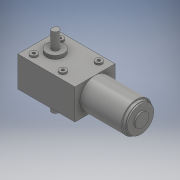
# Autodesk Inventor part: GEARBOX PURNIMA SAMARARATNE
Saved by Autodesk Inventor 2018 (Build 220112000, 112)
## iProperties
Created: 2018-06-19
Part Number: GEARBOX PURNIMA SAMARARATNE
Material: Steel
Document SubType Name: Modeling
Designer: m227958
Density: 7.85 g/cm^3
Appearance: Plate
Author: m227958
Autodesk Inventor part; units mm, degrees
ref_plane "YZ Plane" through (0, 0, 0) normal (1, 0, 0) x (0, 1, 0)
ref_plane "XZ Plane" through (0, 0, 0) normal (0, 1, 0) x (-1, 0, 0)
sketch "Sketch1" plane through (0, 0, 0) normal (1, 0, 0) x (0, 1, 0)
  line L0 (29, 22) -> (-29, 22)
  line L1 (-29, 22) -> (-29, -22)
  line L2 (-29, -22) -> (29, -22)
  line L3 (29, -22) -> (29, 22)
  dimension "d4" = 58
  dimension "d5" = 44
  constraints: 8 end point, 2 parallel, 1 horizontal, 1 perpendicular
  measures "d4" distance of L2.end L1.end
  measures "d5" distance of L1.end L0.end
extrude "Extrusion1" add sketch "Sketch1" along normal blind 82.5
sketch "Sketch2" plane through (82.5, 0, 0) normal (1, 0, 0) x (0, 0, -1)
  circle A0 centre (0, 0) radius 22
  dimension "d8" = 44
  constraints: 1 centre point, 1 coincident
  measures "d8" diameter of A0
extrude "Extrusion2" add sketch "Sketch2" along normal blind 60
sketch "Sketch3" plane through (142.5, 0, 0) normal (1, 0, 0) x (0, 0, -1)
  circle A0 centre (0, 0) radius 20
  dimension "d11" = 40
  constraints: 1 centre point, 1 coincident
  measures "d11" diameter of A0
extrude "Extrusion3" add sketch "Sketch3" along normal blind 4
sketch "Sketch4" plane through (146.5, 0, 0) normal (1, 0, 0) x (0, 0, -1)
  circle A0 centre (0, 0) radius 19
  dimension "d14" = 38
  constraints: 1 centre point, 1 coincident
  measures "d14" diameter of A0
extrude "Extrusion4" add sketch "Sketch4" along normal blind 2
sketch "Sketch5" plane through (148.5, 0, 0) normal (1, 0, 0) x (0, 0, -1)
  circle A0 centre (0, 0) radius 10
  dimension "d17" = 20
  constraints: 1 centre point, 1 coincident
  measures "d17" diameter of A0
extrude "Extrusion5" add sketch "Sketch5" along normal blind 2
sketch "Sketch6" plane through (0, -29, -22) normal (0, 0, -1) x (-1, 0, 0)
  circle A0 centre (-25, 29) radius 12.5
  point P0 (0, 29)
  dimension "d21" = 25
  constraints: 1 centre point
  measures "d21" diameter of A0
extrude "Extrusion6" add sketch "Sketch6" along normal blind 5
sketch "Sketch7" plane through (0, -29, -22) normal (0, 0, -1) x (-1, 0, 0)
  line L0 (0, 0) -> (-82.5, 0) projected
  line L1 (0, 0) -> (0, 58) projected
  circle A0 centre (-13, 10) radius 5
  line L2 (-82.5, 29) -> (-82.5, 58) projected
  circle A1 centre (-13, 48) radius 5
  point P0 (0, 29)
  dimension "d28" = 10
  constraints: 2 centre point
  measures "d28" diameter of A0
extrude "Extrusion7" add sketch "Sketch7" along normal blind 2.5
sketch "Sketch8" plane through (0, -29, -22) normal (0, 0, -1) x (-1, 0, 0)
  line L0 (0, 0) -> (-82.5, 0) projected
  circle A0 centre (-55, 10) radius 5
  point P0 (0, 29)
  dimension "d33" = 10
  constraints: 1 centre point
  measures "d33" diameter of A0
extrude "Extrusion8" add sketch "Sketch8" along normal blind 2.5
sketch "Sketch9" plane through (0, -29, -22) normal (0, 0, -1) x (-1, 0, 0)
  circle A0 centre (-69, 48) radius 5
  point P0 (0, 29)
  point P1 (0, 58)
  dimension "d38" = 10
  constraints: 1 centre point
  measures "d38" diameter of A0
extrude "Extrusion9" add sketch "Sketch9" along normal blind 2.5
sketch "Sketch10" plane through (55, -19, -24.5) normal (0, 0, -1) x (-1, 0, 0)
  circle A0 centre (0, 0) radius 2
  point P0 (55, 19)
  dimension "d41" = 4
  constraints: 1 centre point
  measures "d41" diameter of A0
extrude "Extrusion10" cut sketch "Sketch10" against normal blind 5
sketch "Sketch11" plane through (69, 19, -24.5) normal (0, 0, -1) x (-1, 0, 0)
  circle A0 centre (0, 0) radius 2
  point P0 (69, -19)
  dimension "d44" = 4
  constraints: 1 centre point
  measures "d44" diameter of A0
extrude "Extrusion11" cut sketch "Sketch11" against normal blind 4
sketch "Sketch12" plane through (13, -19, -24.5) normal (0, 0, -1) x (-1, 0, 0)
  circle A0 centre (0, 0) radius 2
  point P0 (13, 19)
  dimension "d47" = 4
  constraints: 1 centre point
  measures "d47" diameter of A0
extrude "Extrusion12" cut sketch "Sketch12" against normal blind 4
sketch "Sketch13" plane through (13, 19, -24.5) normal (0, 0, -1) x (-1, 0, 0)
  circle A0 centre (0, 0) radius 2
  point P0 (13, -19)
  dimension "d50" = 4
  constraints: 1 centre point
  measures "d50" diameter of A0
extrude "Extrusion13" cut sketch "Sketch13" against normal blind 4
sketch "Sketch14" plane through (25, 0, -27) normal (0, 0, -1) x (-1, 0, 0)
  circle A0 centre (0, 0) radius 5
  point P0 (25, 0)
  dimension "d53" = 10
  constraints: 1 centre point
  measures "d53" diameter of A0
extrude "Extrusion14" add sketch "Sketch14" along normal blind 9
sketch "Sketch15" plane through (25, 0, -36) normal (0, 0, -1) x (-1, 0, 0)
  circle A0 centre (0, 0) radius 5 projected
  line L0 (3.5, -3.5707) -> (3.5, 3.5707)
  arc A1 (3.5, 3.5707) -> (3.5, -3.5707) centre (0, 0) ccw
  point P0 (25, 0)
  constraints: 4 point on circle, 2 end point, 1 centre point, 1 concentric
extrude "Extrusion15" add sketch "Sketch15" along normal blind 15 contours L0 A0 picked at (0.6794, -0.2053)
ref_plane "Work Plane1" through (0, -29, 0) normal (0, 0, 1) x (1, 0, 0)
mirror "Mirror1" about plane through (0, -29, 0) normal (0, 0, 1) of "Extrusion8", "Extrusion10", "Extrusion9", "Extrusion11", "Extrusion6", "Extrusion14", "Extrusion15", "Extrusion7", "Extrusion12", "Extrusion13"
equation "\"d45\" = d44"
equation "\"d48\" = d47"
equation "\"d51\" = d50"
body "Solid1"
